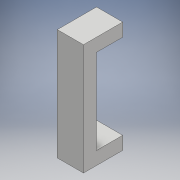
# Autodesk Inventor part: ExtraSupport
Saved by Autodesk Inventor 2017 (Build 210142000, 142)
## iProperties
Created: 2016-11-02
Part Number: ExtraSupport
Material: Generic
Document SubType Name: Modeling
Designer: Schmidty15
Density: 1 g/cm^3
Appearance: Default
Author: Schmidty15
Autodesk Inventor part; units mm, degrees
ref_plane "YZ Plane" through (0, 0, 0) normal (1, 0, 0) x (0, 1, 0)
ref_plane "XZ Plane" through (0, 0, 0) normal (0, 1, 0) x (-1, 0, 0)
ref_plane "XY Plane" through (0, 0, 0) normal (0, 0, 1) x (1, 0, 0)
sketch "Sketch1" plane through (0, 0, 0) normal (0, 1, 0) x (-1, 0, 0)
  line L0 (0, 0) -> (-20, 0)
  line L1 (-20, 0) -> (-20, 85)
  line L2 (-20, 85) -> (0, 85)
  line L3 (0, 85) -> (0, 0)
  dimension "d0" = 20
  dimension "d1" = 85
  constraints: 8 end point, 2 parallel, 1 horizontal, 1 perpendicular
  measures "d0" distance of L1.end L2.end
  measures "d1" distance of L0.end L1.end
extrude "Extrusion1" add sketch "Sketch1" along normal blind 10
sketch "Sketch2" plane through (0, 10, 0) normal (0, 1, 0) x (1, 0, 0)
  line L0 (20, -85) -> (20, 0) projected
  line L1 (0, 0) -> (0, -85) projected
  line L2 (20, 0) -> (0, 0)
  line L3 (0, 0) -> (0, -10)
  line L4 (0, -10) -> (20, -10)
  line L5 (20, -10) -> (20, 0)
  line L6 (0, -85) -> (20, -85) projected
  line L7 (20, -85) -> (0, -85)
  line L8 (0, -85) -> (0, -75)
  line L9 (0, -75) -> (20, -75)
  line L10 (20, -75) -> (20, -85)
  dimension "d4" = 10
  dimension "d5" = 10
  constraints: 16 end point, 4 parallel, 2 horizontal, 2 perpendicular, 2 point on line
  measures "d4" distance of L3.end L2.end
  measures "d5" distance of L7.end L8.end
extrude "Extrusion2" add sketch "Sketch2" along normal blind 20 contours L6 L1 L9 L0 | L4 L1 L2 L0
body "Solid1"
